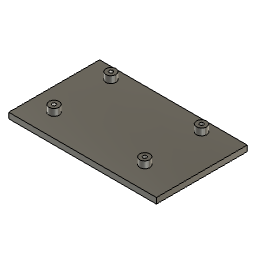
Objectblock Charsiu Board Design v3 (Autodesk Fusion 360 design; units mm, degrees)
Autodesk Fusion 360 part; units mm, degrees
sketch "Sketch1" plane through (0, 0, 0) normal (0, 0, 1) x (1, 0, 0)
  line L0 (0, 0) -> (130, 0)
  line L1 (130, 0) -> (130, 80)
  line L2 (130, 80) -> (0, 80)
  line L3 (0, 80) -> (0, 0)
  dimension "d1" = 130
  dimension "d2" = 80
  constraint horizontal L0
  constraint vertical L1
  constraint horizontal L2
  constraint vertical L3
  constraint coincident L0.start L3.end
  measures "d1" distance of L0.start L0.end
  measures "d2" distance of L0.start L2.end
sketch "Sketch2" plane through (0, 0, 0) normal (0, 0, 1) x (1, 0, 0)
extrude "Extrude1" add sketch "Sketch1" along normal blind 5
sketch "Sketch3" plane through (0, 0, 5) normal (0, 0, 1) x (-1, 0, 0)
  line L0 (0, -80) -> (0, 0)
  line L1 (0, 0) -> (-130, 0)
  line L2 (-130, 0) -> (-130, -80)
  line L3 (-130, -80) -> (0, -80)
  circle A0 centre (-20, -70) radius 4.5
  dimension "d6" = 9
  measures "d6" diameter of A0
extrude "Extrude2" add sketch "Sketch3" along normal blind 6 contours A0
hole "Hole1" at (20, 70, 11) direction (0, 0, -1) diameter 3.783 depth 5.5 tip angle 180
thread "Thread1" "ISO Metric profile 4.5 M4.5x0.75 6H"
sketch "Sketch4" plane through (0, 0, 5) normal (0, 0, 1) x (-1, 0, 0)
  circle A0 centre (-20, -70) radius 4.5
  line L0 (0, -80) -> (0, 0)
  line L1 (0, 0) -> (-130, 0)
  line L2 (-130, 0) -> (-130, -80)
  line L3 (-130, -80) -> (0, -80)
  line L4 (-22, -70) -> (-99.75, -70)
  line L5 (-99.75, -70) -> (-99.75, -69)
  line L6 (-99.75, -69) -> (-22, -69)
  line L7 (-22, -69) -> (-22, -70)
  circle A1 centre (-99.75, -70) radius 4.5
  dimension "d12" = 77.75
  dimension "d13" = 9
  constraint horizontal L4
  constraint vertical L5
  constraint horizontal L6
  constraint vertical L7
  constraint coincident L4.end L5.start
  measures "d12" distance of L4.start L4.end
  measures "d13" diameter of A1
extrude "Extrude3" add sketch "Sketch4" along normal blind 6 contours L4 L5 L6 A1 | L4 L5 L6 A1
delete_face "DeleteFace1" 1 faces at (18.4642, 68.8958, 9.1667)
sketch "Sketch5" plane through (0, 0, 5) normal (0, 0, 1) x (-1, 0, 0)
  circle A0 centre (-99.75, -70) radius 4.5
  circle A1 centre (-20, -70) radius 4.5
  line L0 (0, -80) -> (0, 0)
  line L1 (0, 0) -> (-130, 0)
  line L2 (-130, 0) -> (-130, -80)
  line L3 (-130, -80) -> (0, -80)
  line L4 (-99.8496, -65.5011) -> (-99, -65.5011)
  line L5 (-99, -65.5011) -> (-99, -19.9511)
  line L6 (-99, -19.9511) -> (-99.8496, -19.9511)
  line L7 (-99.8496, -19.9511) -> (-99.8496, -65.5011)
  circle A2 centre (-99.8496, -19.9511) radius 4.5
  dimension "d16" = 45.55
  dimension "d17" = 9
  constraint horizontal L4
  constraint vertical L5
  constraint horizontal L6
  constraint vertical L7
  constraint coincident A0 L4.start
  constraint coincident L6.end L7.start
  measures "d16" distance of L4.start L6.end
  measures "d17" diameter of A2
sketch "Sketch6" plane through (0, 0, 5) normal (0, 0, 1) x (-1, 0, 0)
  line L0 (-19.9427, -65.4909) -> (-21, -65.4909)
  line L1 (-21, -65.4909) -> (-21, -19.9909)
  line L2 (-21, -19.9909) -> (-19.9427, -19.9909)
  line L3 (-19.9427, -19.9909) -> (-19.9427, -65.4909)
  circle A0 centre (-19.9427, -19.9909) radius 4.5
  dimension "d18" = 45.5
  dimension "d19" = 9
  constraint horizontal L0
  constraint vertical L1
  constraint horizontal L2
  constraint vertical L3
  constraint coincident L2.end L3.start
  measures "d18" distance of L0.start L2.end
  measures "d19" diameter of A0
extrude "Extrude4" add sketch "Sketch5" sketch "Sketch6" along normal blind 6 contours L5 L6 L7 A2 | L5 L6 L7 A2 of sketch 2 contours L1 L2 L3 A0 | L1 L2 L3 A0
hole "Hole2" at (99.8496, 19.9511, 11) direction (0, 0, -1) diameter 3.332 depth 5 tip angle 180
thread "Thread2" "ISO Metric profile 4.0 M4x0.7 6H"
hole "Hole3" at (99.75, 70, 11) direction (0, 0, -1) diameter 3.332 depth 5 tip angle 180
thread "Thread3" "ISO Metric profile 4.0 M4x0.7 6H" major diameter 4.1095 minor diameter 3.332 pitch 0.7 angle 60 resizes the face on face at (98.5009, 68.8976, 9.3333)
hole "Hole4" at (19.9427, 19.9909, 11) direction (0, 0, -1) diameter 3.332 depth 5 tip angle 180
thread "Thread4" "ISO Metric profile 4.0 M4x0.7 6H"
hole "Hole5" at (20, 70, 11) direction (0, 0, -1) diameter 3.332 depth 5 tip angle 180
thread "Thread5" "ISO Metric profile 4.0 M4x0.7 6H"
